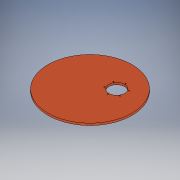
# Autodesk Inventor part: 2K8 stage
Saved by Autodesk Inventor 2018 (Build 220112000, 112)
## iProperties
Created: 2018-10-14
Part Number: 2K8 stage
Material: Copper
Document SubType Name: Modeling
Designer: freyja
Mass: 11045.9 g
Surface Area: 2715.95 cm^2
Volume: 1235.56 cm^3
Density: 8.94 g/cm^3
Appearance: Copper - Satin
Author: freyja
Autodesk Inventor part; units mm, degrees
note: some values were not read from the file. Chosen so that the rebuilt part matches the saved one: direction of "Hole1".
ref_plane "YZ Plane" through (0, 0, 0) normal (1, 0, 0) x (0, 1, 0)
ref_plane "XZ Plane" through (0, 0, 0) normal (0, 1, 0) x (-1, 0, 0)
ref_plane "XY Plane" through (0, 0, 0) normal (0, 0, 1) x (1, 0, 0)
sketch "Sketch1" plane through (0, 0, 0) normal (0, 1, 0) x (-1, 0, 0)
  circle A0 centre (0, 0) radius 203.2
  dimension "d0" = 406.4
  constraints: 1 centre point, 1 coincident
  measures "d0" diameter of A0
extrude "Extrusion1" add sketch "Sketch1" along normal blind 9.525
sketch "Sketch2" plane through (0, 9.525, 0) normal (0, 1, 0) x (1, 0, 0)
  line L0 (0, 0) -> (64.6578, 64.6578) construction
  line L1 (0, 0) -> (91.44, 0) construction
  line L2 (64.6578, 64.6578) -> (102.0528, 86.2478)
  line L3 (64.6578, 64.6578) -> (107.8378, 64.6578) construction
  line L4 (64.6578, 64.6578) -> (64.6578, 107.8378)
  line L5 (64.6578, 64.6578) -> (27.2629, 86.2478)
  line L6 (64.6578, 64.6578) -> (27.2629, 43.0678)
  line L7 (64.6578, 64.6578) -> (64.6578, 21.4778)
  line L8 (64.6578, 64.6578) -> (102.0528, 43.0678)
  dimension "d3" = 91.44
  dimension "d4" = 45
  dimension "d5" = 43.18
  dimension "d6" = 30
  dimension "d9" = 360
  constraints: 18 end point, 2 coincident, 2 equal length, 2 horizontal, 17 other
  measures "d3" distance of L0.start L0.end
  measures "d4" angle of L1 L0
  measures "d5" distance of L0.end L2.end
  measures "d6" angle of L3 L2
hole "Hole1" at (64.6578, 9.525, -107.8378) at (27.2629, 9.525, -86.2478) at (27.2629, 9.525, -43.0678) at (102.0528, 9.525, -43.0678) at (102.0528, 9.525, -86.2478) at (64.6578, 9.525, -21.4778) direction (0, -1, 0) diameter 4.1402 end up to surface
sketch "Sketch3" plane through (0, 9.525, 0) normal (0, 1, 0) x (1, 0, 0)
  line L0 (0, 0) -> (64.6578, 64.6578) construction
  line L1 (0, 0) -> (91.44, 0) construction
  circle A0 centre (64.6578, 64.6578) radius 38.1
  dimension "d18" = 91.44
  dimension "d19" = 45
  dimension "d20" = 76.2
  constraints: 4 end point, 1 centre point, 1 coincident, 1 equal length, 1 horizontal
  measures "d18" distance of L0.start L0.end
  measures "d19" angle of L1 L0
  measures "d20" diameter of A0
extrude "Extrusion2" cut sketch "Sketch3" against normal up to surface (9.525 mm away)
body "Solid1"
